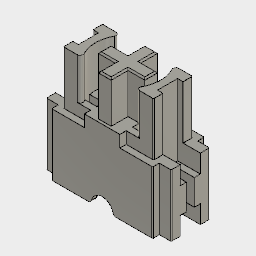
ALPS to MX stem (Autodesk Fusion 360 design; units mm, degrees)
Autodesk Fusion 360 part; units mm, degrees
sketch "Sketch1" plane through (0, 0, 0) normal (0, 0, 1) x (1, 0, 0)
  line L0 (0, 0) -> (10.7188, 0)
  line L1 (10.7188, 0) -> (10.7188, 4.445)
  line L2 (10.7188, 4.445) -> (0, 4.445)
  line L3 (0, 4.445) -> (0, 0)
  line L4 (0, 4.445) -> (1.016, 4.445)
  line L5 (1.016, 4.445) -> (1.016, 3.8735)
  line L6 (1.016, 3.8735) -> (0, 3.8735)
  line L7 (0, 3.8735) -> (0, 4.445)
  line L8 (0, 0) -> (1.016, 0)
  line L9 (1.016, 0) -> (1.016, 0.5715)
  line L10 (1.016, 0.5715) -> (0, 0.5715)
  line L11 (0, 0.5715) -> (0, 0)
  line L12 (10.7188, 4.445) -> (9.7028, 4.445)
  line L13 (9.7028, 4.445) -> (9.7028, 3.8735)
  line L14 (9.7028, 3.8735) -> (10.7188, 3.8735)
  line L15 (10.7188, 3.8735) -> (10.7188, 4.445)
  line L16 (10.7188, 0) -> (9.7028, 0)
  line L17 (9.7028, 0) -> (9.7028, 0.5715)
  line L18 (9.7028, 0.5715) -> (10.7188, 0.5715)
  line L19 (10.7188, 0.5715) -> (10.7188, 0)
  line L20 (5.3594, 4.445) -> (5.3594, 0) construction
  line L21 (0, 2.2225) -> (10.7188, 2.2225) construction
  line L22 (0, 3.0861) -> (1.9558, 3.0861)
  line L23 (1.9558, 3.0861) -> (1.9558, 1.3589)
  line L24 (1.9558, 1.3589) -> (0, 1.3589)
  line L25 (0, 1.3589) -> (0, 3.0861)
  line L26 (8.763, 3.0861) -> (10.7188, 3.0861)
  line L27 (10.7188, 3.0861) -> (10.7188, 1.3589)
  line L28 (10.7188, 1.3589) -> (8.763, 1.3589)
  line L29 (8.763, 1.3589) -> (8.763, 3.0861)
  circle A0 centre (5.3594, 2.2225) radius 1.0922
  circle A1 centre (5.3594, 2.2225) radius 1.905
  line L30 (1.9558, 3.0861) -> (2.5908, 3.0861)
  line L31 (2.5908, 3.0861) -> (2.5908, 1.3589)
  line L32 (2.5908, 1.3589) -> (1.9558, 1.3589)
  line L33 (1.9558, 1.3589) -> (1.9558, 3.0861)
  line L34 (8.763, 3.0861) -> (8.128, 3.0861)
  line L35 (8.128, 3.0861) -> (8.128, 1.3589)
  line L36 (8.128, 1.3589) -> (8.763, 1.3589)
  line L37 (8.763, 1.3589) -> (8.763, 3.0861)
  line L38 (2.5908, 3.3655) -> (3.8354, 3.3655)
  line L39 (3.8354, 3.3655) -> (3.8354, 1.0795)
  line L40 (3.8354, 1.0795) -> (2.5908, 1.0795)
  line L41 (2.5908, 1.0795) -> (2.5908, 3.3655)
  line L42 (8.128, 3.3655) -> (6.8834, 3.3655)
  line L43 (6.8834, 3.3655) -> (6.8834, 1.0795)
  line L44 (6.8834, 1.0795) -> (8.128, 1.0795)
  line L45 (8.128, 1.0795) -> (8.128, 3.3655)
  dimension "d1" = 4.445
  dimension "d2" = 10.7188
  dimension "d3" = 3.302
  dimension "d4" = 1.7272
  dimension "d5" = 8.6868
  dimension "d6" = 6.8072
  dimension "d7" = 2.1844
  dimension "d8" = 3.81
  dimension "d10" = 0.635
  dimension "d12" = 2.286
  measures "d1" distance of L0.start L2.end
  measures "d2" distance of L1.end L2.end
  measures "d3" distance of L6 L10
  measures "d4" distance of L22.end L23.end
  measures "d5" distance of L5 L13
  measures "d6" distance of L23 L29
  measures "d7" diameter of A0
  measures "d8" diameter of A1
  measures "d10" distance of L22.end L30.end
  measures "d12" distance of L38.start L40.end
extrude "Extrude1" add sketch "Sketch1" along normal blind 5.334 contours L0 L1 L3 L9 L10 L17 L18 L24 L28 A1 L32 L36 L40 L41 L44 L45 | L1 L2 L3 L5 L6 L13 L14 L22 L26 A1 L30 L34 L38 L41 L42 L45 | L23 L30 L31 L32 L33 L41 | L29 L34 L35 L36 L37 L45 | A0 makes body 1 at (6.4502, 2.1681, 3.556) makes body 2 at (3.9116, 4.445, 3.556)
sketch "Sketch2" plane through (0, 0, 0) normal (-1, 0, 0) x (0, -1, 0)
  line L0 (-1.3589, 0) -> (-0.5715, 0) construction
  line L1 (-0.5715, 0) -> (-0.5715, 5.334) construction
  line L2 (-0.5715, 5.334) -> (-1.3589, 5.334) construction
  line L3 (-1.3589, 5.334) -> (-1.3589, 0) construction
  line L4 (-1.3589, 5.334) -> (-0.5715, 5.334) construction
  line L5 (-3.8735, 5.334) -> (-3.0861, 5.334) construction
  line L6 (-3.8735, 5.334) -> (-3.0861, 5.334) construction
  line L7 (-3.0861, 5.334) -> (-3.0861, 0) construction
  line L8 (-3.0861, 0) -> (-3.8735, 0) construction
  line L9 (-3.8735, 0) -> (-3.8735, 5.334) construction
  line L10 (-1.3589, 5.334) -> (-0.5715, 5.334) construction
  line L11 (-0.5715, 5.334) -> (-0.5715, 0) construction
  line L12 (-0.5715, 0) -> (-1.3589, 0) construction
  line L13 (-1.3589, 0) -> (-1.3589, 5.334) construction
  line L14 (-3.8735, 2.667) -> (-0.5715, 2.667) construction
  line L15 (-3.0861, 3.7719) -> (-2.5654, 3.7719)
  line L16 (-2.5654, 3.7719) -> (-2.5654, 1.5621)
  line L17 (-2.5654, 1.5621) -> (-3.0861, 1.5621)
  line L18 (-3.0861, 1.5621) -> (-3.0861, 3.7719)
  line L19 (-1.3589, 3.7719) -> (-1.8796, 3.7719)
  line L20 (-1.8796, 3.7719) -> (-1.8796, 1.5621)
  line L21 (-1.8796, 1.5621) -> (-1.3589, 1.5621)
  line L22 (-1.3589, 1.5621) -> (-1.3589, 3.7719)
  point P0 (-3.0861, 0)
  dimension "d16" = 2.2098
  dimension "d17" = 0.6858
  dimension "d18" = 1.3081
  measures "d16" distance of L15 L17
  measures "d17" distance of L16 L20
  measures "d18" distance of L9 L16
extrude "Extrude2" add sketch "Sketch2" against normal up to surface (1.9558 mm away) bodies 2
sketch "Sketch3" plane through (10.7188, 0, 0) normal (1, 0, 0) x (0, 1, 0)
  line L0 (0.5715, 0) -> (1.3589, 0)
  line L1 (1.3589, 0) -> (1.3589, 5.334)
  line L2 (1.3589, 5.334) -> (0.5715, 5.334)
  line L3 (0.5715, 5.334) -> (0.5715, 0)
  line L4 (3.8735, 0) -> (3.0861, 0)
  line L5 (3.0861, 0) -> (3.0861, 1.5621)
  line L6 (3.0861, 1.5621) -> (2.5654, 1.5621)
  line L7 (2.5654, 1.5621) -> (2.5654, 3.7719)
  line L8 (2.5654, 3.7719) -> (3.0861, 3.7719)
  line L9 (3.0861, 3.7719) -> (3.0861, 5.334)
  line L10 (3.0861, 5.334) -> (3.8735, 5.334)
  line L11 (3.8735, 5.334) -> (3.8735, 0)
  line L12 (1.3589, 0) -> (0.5715, 0)
  line L13 (0.5715, 0) -> (0.5715, 5.334)
  line L14 (0.5715, 5.334) -> (1.3589, 5.334)
  line L15 (1.3589, 5.334) -> (1.3589, 3.7719)
  line L16 (1.3589, 3.7719) -> (1.8796, 3.7719)
  line L17 (1.8796, 3.7719) -> (1.8796, 1.5621)
  line L18 (1.8796, 1.5621) -> (1.3589, 1.5621)
  line L19 (1.3589, 1.5621) -> (1.3589, 0)
  line L20 (3.0861, 3.7719) -> (3.0861, 1.5621)
  line L21 (1.3589, 3.7719) -> (1.3589, 1.5621)
extrude "Extrude3" add sketch "Sketch3" against normal up to surface (1.9558 mm away) contours L1 L16 L17 L18 L21 | L6 L7 L8 L20 bodies 2
sketch "Sketch4" plane through (0, 0, 5.334) normal (0, 0, 1) x (-1, 0, 0)
  arc A0 (-3.8354, -1.0795) -> (-6.8834, -1.0795) centre (-5.3594, -2.2225) ccw
  line L0 (-3.8354, -1.0795) -> (-2.5908, -1.0795)
  line L1 (-2.5908, -1.0795) -> (-2.5908, -3.3655)
  line L2 (-2.5908, -3.3655) -> (-3.8354, -3.3655)
  arc A1 (-6.8834, -3.3655) -> (-3.8354, -3.3655) centre (-5.3594, -2.2225) ccw
  line L3 (-6.8834, -3.3655) -> (-8.128, -3.3655)
  line L4 (-8.128, -3.3655) -> (-8.128, -1.0795)
  line L5 (-8.128, -1.0795) -> (-6.8834, -1.0795)
  line L6 (-1.016, 0) -> (-9.7028, 0)
  line L7 (-9.7028, 0) -> (-9.7028, -0.5715)
  line L8 (-9.7028, -0.5715) -> (-10.7188, -0.5715)
  line L9 (-10.7188, -0.5715) -> (-10.7188, -1.3589)
  line L10 (-10.7188, -1.3589) -> (-8.763, -1.3589)
  line L11 (-8.763, -1.3589) -> (-8.763, -3.0861)
  line L12 (-8.763, -3.0861) -> (-10.7188, -3.0861)
  line L13 (-10.7188, -3.0861) -> (-10.7188, -3.8735)
  line L14 (-10.7188, -3.8735) -> (-9.7028, -3.8735)
  line L15 (-9.7028, -3.8735) -> (-9.7028, -4.445)
  line L16 (-9.7028, -4.445) -> (-1.016, -4.445)
  line L17 (-1.016, -4.445) -> (-1.016, -3.8735)
  line L18 (-1.016, -3.8735) -> (0, -3.8735)
  line L19 (0, -3.8735) -> (0, -3.0861)
  line L20 (0, -3.0861) -> (-1.9558, -3.0861)
  line L21 (-1.9558, -3.0861) -> (-1.9558, -1.3589)
  line L22 (-1.9558, -1.3589) -> (0, -1.3589)
  line L23 (0, -1.3589) -> (0, -0.5715)
  line L24 (0, -0.5715) -> (-1.016, -0.5715)
  line L25 (-1.016, -0.5715) -> (-1.016, 0)
  circle A2 centre (-5.3594, -2.2225) radius 1.0922
  line L26 (-5.9055, -4.2164) -> (-4.8133, -4.2164)
  line L27 (-4.8133, -4.2164) -> (-4.8133, -0.2286)
  line L28 (-4.8133, -0.2286) -> (-5.9055, -0.2286)
  line L29 (-5.9055, -0.2286) -> (-5.9055, -4.2164)
  line L30 (-5.9055, -4.2164) -> (-4.8133, -0.2286) construction
  line L31 (-4.8133, -4.2164) -> (-5.9055, -0.2286) construction
  line L32 (-7.3533, -2.7686) -> (-3.3655, -2.7686)
  line L33 (-3.3655, -2.7686) -> (-3.3655, -1.6764)
  line L34 (-3.3655, -1.6764) -> (-7.3533, -1.6764)
  line L35 (-7.3533, -1.6764) -> (-7.3533, -2.7686)
  line L36 (-7.3533, -2.7686) -> (-3.3655, -1.6764) construction
  line L37 (-3.3655, -2.7686) -> (-7.3533, -1.6764) construction
  line L38 (-6.8834, -4.445) -> (-3.8354, -4.445)
  line L39 (-3.8354, -4.445) -> (-3.8354, 0)
  line L40 (-3.8354, 0) -> (-6.8834, 0)
  line L41 (-6.8834, 0) -> (-6.8834, -4.445)
  line L42 (-6.8834, -4.445) -> (-3.8354, 0) construction
  line L43 (-3.8354, -4.445) -> (-6.8834, 0) construction
  line L44 (-3.3655, -2.7686) -> (-1.9558, -2.7686)
  line L45 (-1.9558, -2.7686) -> (-1.9558, -1.6764)
  line L46 (-1.9558, -1.6764) -> (-3.3655, -1.6764)
  line L47 (-3.3655, -1.6764) -> (-3.3655, -2.7686)
  line L48 (-7.3533, -2.7686) -> (-8.763, -2.7686)
  line L49 (-8.763, -2.7686) -> (-8.763, -1.6764)
  line L50 (-8.763, -1.6764) -> (-7.3533, -1.6764)
  line L51 (-7.3533, -1.6764) -> (-7.3533, -2.7686)
  point P0 (-5.3594, -2.2225)
  point P1 (-5.3594, -2.2225)
  point P2 (-5.3594, -2.2225)
  dimension "d23" = 1.0922
  dimension "d25" = 3.9878
  measures "d23" distance of L26.start L26.end
  measures "d25" distance of L26.start L28.end
extrude "Extrude4" add sketch "Sketch4" along normal blind 1.016 contours A0 A2 L27 L34 L39 | A0 L6 L27 L28 L29 L39 L40 L41 | A0 A2 L27 L29 | A0 L27 L28 L29 | A2 L32 L34 L39 | L32 L33 L34 L39 L47 | A0 A2 L29 L34 L41 | A2 L27 L29 L34 | A2 L27 L34 | L1 L21 L44 L45 L46 | L1 L33 L44 L46 L47 | A2 L27 L32 L34 | A1 A2 L27 L32 L39 | A2 L29 L34 | L27 L29 L32 L34 | A2 L27 L32 | A1 L16 L26 L27 L29 L38 L39 L41 | L32 L34 L35 L41 L51 | A2 L32 L34 L41 | A2 L29 L32 L34 | A2 L27 L29 L32 | A1 A2 L27 L29 | A1 L26 L27 L29 | L4 L35 L48 L50 L51 | L4 L11 L48 L49 L50 | A1 A2 L29 L32 L41 | A2 L29 L32 bodies 1 2
sketch "Sketch5" plane through (0, 0, 6.35) normal (0, 0, 1) x (-1, 0, 0)
  line L0 (-6.8834, 0) -> (-6.8834, -1.6764)
  line L1 (-6.8834, -4.445) -> (-3.8354, -4.445)
  line L2 (-3.8354, -4.445) -> (-3.8354, -2.7686)
  line L3 (-3.8354, 0) -> (-6.8834, 0)
  line L4 (-3.3655, -2.7686) -> (-3.3655, -1.6764)
  line L5 (-7.3533, -2.7686) -> (-3.3655, -2.7686)
  line L6 (-3.3655, -1.6764) -> (-7.3533, -1.6764)
  line L7 (-7.3533, -1.6764) -> (-7.3533, -2.7686)
  line L8 (-5.9055, -0.2286) -> (-5.9055, -4.2164)
  line L9 (-5.9055, -4.2164) -> (-4.8133, -4.2164)
  line L10 (-4.8133, -4.2164) -> (-4.8133, -0.2286)
  line L11 (-4.8133, -0.2286) -> (-5.9055, -0.2286)
  line L12 (-6.8834, -1.6764) -> (-8.763, -1.6764)
  line L13 (-8.763, -2.7686) -> (-6.8834, -2.7686)
  line L14 (-6.8834, -2.7686) -> (-6.8834, -4.445)
  line L15 (-3.8354, -2.7686) -> (-1.9558, -2.7686)
  line L16 (-1.9558, -1.6764) -> (-3.8354, -1.6764)
  line L17 (-3.8354, -1.6764) -> (-3.8354, 0)
  line L18 (-1.9558, -2.7686) -> (-1.9558, -1.6764)
  line L19 (-8.763, -1.6764) -> (-8.763, -2.7686)
extrude "Extrude5" add sketch "Sketch5" along normal blind 3.556 contours L5 L6 L7 L8 L12 L13 | L6 L8 L10 L11 | L5 L6 L8 L10 | L4 L5 L6 L10 L15 L16 | L5 L8 L9 L10 bodies 1
sketch "Sketch6" plane through (0, 0, 5.334) normal (0, 0, 1) x (-1, 0, 0)
  line L0 (-8.763, -1.6764) -> (-8.128, -1.6764)
  line L1 (-8.128, -1.6764) -> (-8.128, -1.0795)
  line L2 (-8.128, -1.0795) -> (-6.8834, -1.0795)
  line L3 (-6.8834, -1.0795) -> (-6.8834, 0)
  line L4 (-6.8834, 0) -> (-9.7028, 0)
  line L5 (-9.7028, 0) -> (-9.7028, -0.5715)
  line L6 (-9.7028, -0.5715) -> (-10.7188, -0.5715)
  line L7 (-10.7188, -0.5715) -> (-10.7188, -1.3589)
  line L8 (-10.7188, -1.3589) -> (-8.763, -1.3589)
  line L9 (-8.763, -1.3589) -> (-8.763, -1.6764)
  line L10 (-6.8834, -4.445) -> (-6.8834, -3.3655)
  line L11 (-6.8834, -3.3655) -> (-8.128, -3.3655)
  line L12 (-8.128, -3.3655) -> (-8.128, -2.7686)
  line L13 (-8.128, -2.7686) -> (-8.763, -2.7686)
  line L14 (-8.763, -2.7686) -> (-8.763, -3.0861)
  line L15 (-8.763, -3.0861) -> (-10.7188, -3.0861)
  line L16 (-10.7188, -3.0861) -> (-10.7188, -3.8735)
  line L17 (-10.7188, -3.8735) -> (-9.7028, -3.8735)
  line L18 (-9.7028, -3.8735) -> (-9.7028, -4.445)
  line L19 (-9.7028, -4.445) -> (-6.8834, -4.445)
  arc A0 (-3.8354, -1.0795) -> (-6.8834, -1.0795) centre (-5.3594, -2.2225) ccw
  line L20 (-6.8834, -1.0795) -> (-8.128, -1.0795)
  line L21 (-8.128, -1.0795) -> (-8.128, -3.3655)
  line L22 (-8.128, -3.3655) -> (-6.8834, -3.3655)
  arc A1 (-6.8834, -3.3655) -> (-3.8354, -3.3655) centre (-5.3594, -2.2225) ccw
  line L23 (-3.8354, -3.3655) -> (-2.5908, -3.3655)
  line L24 (-2.5908, -3.3655) -> (-2.5908, -1.0795)
  line L25 (-2.5908, -1.0795) -> (-3.8354, -1.0795)
  line L26 (-9.7028, 0) -> (-1.016, 0)
  line L27 (-1.016, 0) -> (-1.016, -0.5715)
  line L28 (-1.016, -0.5715) -> (0, -0.5715)
  line L29 (0, -0.5715) -> (0, -1.3589)
  line L30 (0, -1.3589) -> (-1.9558, -1.3589)
  line L31 (-1.9558, -1.3589) -> (-1.9558, -3.0861)
  line L32 (-1.9558, -3.0861) -> (0, -3.0861)
  line L33 (0, -3.0861) -> (0, -3.8735)
  line L34 (0, -3.8735) -> (-1.016, -3.8735)
  line L35 (-1.016, -3.8735) -> (-1.016, -4.445)
  line L36 (-1.016, -4.445) -> (-9.7028, -4.445)
  line L37 (-9.7028, -4.445) -> (-9.7028, -3.8735)
  line L38 (-9.7028, -3.8735) -> (-10.7188, -3.8735)
  line L39 (-10.7188, -3.8735) -> (-10.7188, -3.0861)
  line L40 (-10.7188, -3.0861) -> (-8.763, -3.0861)
  line L41 (-8.763, -3.0861) -> (-8.763, -1.3589)
  line L42 (-8.763, -1.3589) -> (-10.7188, -1.3589)
  line L43 (-10.7188, -1.3589) -> (-10.7188, -0.5715)
  line L44 (-10.7188, -0.5715) -> (-9.7028, -0.5715)
  line L45 (-9.7028, -0.5715) -> (-9.7028, 0)
  line L46 (-5.3594, -4.445) -> (-5.3594, 0) construction
  line L47 (-1.9558, -2.2225) -> (-8.763, -2.2225) construction
  line L48 (-9.2329, -3.8989) -> (-1.4859, -3.8989)
  line L49 (-1.4859, -3.8989) -> (-1.4859, -0.5461)
  line L50 (-1.4859, -0.5461) -> (-9.2329, -0.5461)
  line L51 (-9.2329, -0.5461) -> (-9.2329, -3.8989)
  line L52 (-9.2329, -3.8989) -> (-1.4859, -0.5461) construction
  line L53 (-1.4859, -3.8989) -> (-9.2329, -0.5461) construction
  line L54 (-1.4859, -3.0861) -> (-1.9558, -3.0861)
  line L55 (-1.9558, -3.0861) -> (-1.9558, -1.3589)
  line L56 (-1.9558, -1.3589) -> (-1.4859, -1.3589)
  line L57 (-1.4859, -1.3589) -> (-1.4859, -3.0861)
  circle A2 centre (-5.3594, -2.2225) radius 2.794
  point P0 (-5.3594, -2.2225)
  dimension "d30" = 7.747
  dimension "d31" = 3.3528
  dimension "d32" = 5.588
  measures "d30" distance of L48.start L48.end
  measures "d31" distance of L48.end L49.end
  measures "d32" diameter of A2
extrude "Extrude6" add sketch "Sketch6" along normal up to surface (4.572 mm away) contours L0 L1 L2 L8 L9 L20 L21 L41 L42 L50 L51 A2 | L0 L13 L21 L41 A2 | L1 L2 L20 L21 A2 | L11 L12 L13 L14 L15 L21 L22 L40 L41 L48 L51 A2 | L11 L12 L21 L22 A2 | L23 L24 L25 L30 L31 L32 L48 L49 L50 L54 L55 L56 A2 | L24 L25 A2 | L23 L24 A2 bodies 1
extrude "Extrude7" add sketch "Sketch6" along normal up to surface (1.016 mm away) contours L2 L3 L20 L50 A2 | L10 L11 L22 L48 A2 | A0 L25 L50 A2 | A1 L23 L48 A2 bodies 1
chamfer "Chamfer1" distance 0.127 angle 45 12 edges at (5.3594, 0.2286, 9.906) (3.3655, 2.2225, 9.906) (5.3594, 4.2164, 9.906) (7.3533, 2.2225, 9.906) (6.6294, 1.6764, 9.906) (5.9055, 0.9525, 9.906) (4.8133, 0.9525, 9.906) (4.0894, 1.6764, 9.906) (4.0894, 2.7686, 9.906) (4.8133, 3.4925, 9.906) (5.9055, 3.4925, 9.906) (6.6294, 2.7686, 9.906) on bodies 1
fillet "Fillet1" radius 0.254 4 edges at (3.1242, 0.5461, 8.128) (3.1242, 3.8989, 8.128) (7.5946, 0.5461, 8.128) (7.5946, 3.8989, 8.128) on bodies 1
fillet "Fillet2" radius 0.0762 16 edges at (1.4859, 3.0861, 7.62) (1.4859, 3.8989, 7.62) (1.4859, 1.3589, 7.62) (1.4859, 0.5461, 7.62) (9.2329, 0.5461, 7.62) (9.2329, 1.3589, 7.62) (9.2329, 3.0861, 7.62) (9.2329, 3.8989, 7.62) (1.016, 0, 2.667) (0, 0.5715, 2.667) (0, 3.8735, 2.667) (9.7028, 0, 2.667) (10.7188, 0.5715, 2.667) (10.7188, 3.8735, 2.667) (9.7028, 4.445, 2.667) (1.016, 4.445, 2.667) on bodies 1
fillet "Fillet3" radius 0.127 1 edges at (4.3411, 1.8275, 0) on bodies 1
sketch "Sketch7" plane through (0, 0, 0) normal (0, 0, -1) x (1, 0, 0)
  arc A0 (1.016, -4.3688) -> (1.0922, -4.445) centre (1.0922, -4.3688) ccw
  line L0 (1.0922, -4.445) -> (9.6266, -4.445)
  arc A1 (9.6266, -4.445) -> (9.7028, -4.3688) centre (9.6266, -4.3688) ccw
  line L1 (9.7028, -4.3688) -> (9.7028, -3.8735)
  line L2 (9.7028, -3.8735) -> (10.6426, -3.8735)
  arc A2 (10.6426, -3.8735) -> (10.7188, -3.7973) centre (10.6426, -3.7973) ccw
  line L3 (10.7188, -3.7973) -> (10.7188, -3.0861)
  line L4 (10.7188, -3.0861) -> (8.763, -3.0861)
  line L5 (8.763, -3.0861) -> (8.763, -1.3589)
  line L6 (8.763, -1.3589) -> (10.7188, -1.3589)
  line L7 (10.7188, -1.3589) -> (10.7188, -0.6477)
  arc A3 (10.7188, -0.6477) -> (10.6426, -0.5715) centre (10.6426, -0.6477) ccw
  line L8 (10.6426, -0.5715) -> (9.7028, -0.5715)
  line L9 (9.7028, -0.5715) -> (9.7028, -0.0762)
  arc A4 (9.7028, -0.0762) -> (9.6266, 0) centre (9.6266, -0.0762) ccw
  line L10 (9.6266, 0) -> (1.0922, 0)
  arc A5 (1.0922, 0) -> (1.016, -0.0762) centre (1.0922, -0.0762) ccw
  line L11 (1.016, -0.0762) -> (1.016, -0.5715)
  line L12 (1.016, -0.5715) -> (0.0762, -0.5715)
  arc A6 (0.0762, -0.5715) -> (0, -0.6477) centre (0.0762, -0.6477) ccw
  line L13 (0, -0.6477) -> (0, -1.3589)
  line L14 (0, -1.3589) -> (1.9558, -1.3589)
  line L15 (1.9558, -1.3589) -> (1.9558, -3.0861)
  line L16 (1.9558, -3.0861) -> (0, -3.0861)
  line L17 (0, -3.0861) -> (0, -3.7973)
  arc A7 (0, -3.7973) -> (0.0762, -3.8735) centre (0.0762, -3.7973) ccw
  line L18 (0.0762, -3.8735) -> (1.016, -3.8735)
  line L19 (1.016, -3.8735) -> (1.016, -4.3688)
  arc A8 (6.8834, -1.0795) -> (3.8354, -1.0795) centre (5.3594, -2.2225) ccw
  line L20 (6.8834, -1.0795) -> (8.128, -1.0795)
  line L21 (8.128, -1.0795) -> (8.128, -3.3655)
  line L22 (8.128, -3.3655) -> (6.8834, -3.3655)
  arc A9 (3.8354, -3.3655) -> (6.8834, -3.3655) centre (5.3594, -2.2225) ccw
  line L23 (3.8354, -3.3655) -> (2.5908, -3.3655)
  line L24 (2.5908, -3.3655) -> (2.5908, -1.0795)
  line L25 (2.5908, -1.0795) -> (3.8354, -1.0795)
  line L26 (6.3119, 0) -> (4.4069, 0)
  line L27 (4.4069, 0) -> (4.4069, -4.445)
  line L28 (4.4069, -4.445) -> (6.3119, -4.445)
  line L29 (6.3119, -4.445) -> (6.3119, 0)
  line L30 (6.3119, 0) -> (4.4069, -4.445) construction
  line L31 (4.4069, 0) -> (6.3119, -4.445) construction
  point P0 (5.3594, -2.2225)
  dimension "d42" = 1.905
  measures "d42" distance of L26.start L26.end
sketch "Sketch8" plane through (0, 4.445, 0) normal (0, 1, 0) x (-1, 0, 0)
  line L0 (-1.0922, 0) -> (-1.0922, 5.334)
  line L1 (-1.0922, 5.334) -> (-3.8354, 5.334)
  line L2 (-3.8354, 5.334) -> (-3.8354, 6.35)
  line L3 (-3.8354, 6.35) -> (-6.8834, 6.35)
  line L4 (-6.8834, 6.35) -> (-6.8834, 5.334)
  line L5 (-6.8834, 5.334) -> (-9.6266, 5.334)
  line L6 (-9.6266, 5.334) -> (-9.6266, 0)
  line L7 (-9.6266, 0) -> (-1.0922, 0)
  line L8 (-4.4069, 0) -> (-6.3119, 0)
  circle A0 centre (-5.3594, 0) radius 0.9525
  point P0 (-6.3119, 0)
extrude "Extrude8" cut sketch "Sketch8" against normal blind 0.762 contours L7 L8 A0 picked at (-5.1267, 0.216) bodies 1
sketch "Sketch9" plane through (0, 0, 0) normal (0, -1, 0) x (1, 0, 0)
  line L0 (9.6266, 0) -> (9.6266, 5.334)
  line L1 (9.6266, 5.334) -> (6.8834, 5.334)
  line L2 (6.8834, 5.334) -> (6.8834, 6.35)
  line L3 (6.8834, 6.35) -> (3.8354, 6.35)
  line L4 (3.8354, 6.35) -> (3.8354, 5.334)
  line L5 (3.8354, 5.334) -> (1.0922, 5.334)
  line L6 (1.0922, 5.334) -> (1.0922, 0)
  line L7 (1.0922, 0) -> (9.6266, 0)
  circle A0 centre (5.3594, 0) radius 0.9525
  point P0 (5.3594, 0)
  point P1 (6.3119, 0)
extrude "Extrude9" cut sketch "Sketch9" against normal blind 0.762 contours L7 A0 picked at (5.5921, 0.216) bodies 1
fillet "Fillet4" radius 0.254 4 edges at (6.3119, 0.2864, 0) (4.4069, 0.2864, 0) (4.4069, 4.1586, 0) (6.3119, 4.1586, 0) on bodies 1
fillet "Fillet5" radius 0.254 10 edges at (3.9962, 3.5532, 0) (4.3313, 3.8263, 0.0501) (5.3594, 4.1275, 0.9525) (6.3875, 3.8263, 0.0501) (6.7226, 3.5532, 0) (3.9962, 0.8918, 0) (4.3313, 0.6187, 0.0501) (5.3594, 0.3175, 0.9525) (6.3875, 0.6187, 0.0501) (6.7226, 0.8918, 0) on bodies 1
ref_plane "WorkPlane1" through (0.9779, 2.2225, 2.667) normal (0, -1, 0) x (0, 0, -1)
sketch "Sketch10" plane through (0.9779, 2.2225, 2.667) normal (0, -1, 0) x (1, 0, 0)
  line L0 (5.4737, 2.667) -> (3.2893, 2.667)
  line L1 (3.2893, -2.54) -> (5.4737, -2.54)
  line L2 (7.1501, -2.667) -> (7.1501, 2.667)
  line L3 (1.6129, -2.667) -> (1.6129, 2.667)
  line L4 (1.6129, 2.667) -> (1.6129, -2.667)
  line L5 (5.4737, 2.667) -> (7.1501, 2.2178)
  line L6 (3.2893, 2.667) -> (1.6129, 2.2178)
  line L7 (2.8575, 2.667) -> (1.6414, 2.667)
  line L8 (5.9055, 2.667) -> (7.1216, 2.667)
  line L9 (7.1501, 2.2178) -> (7.1501, 2.667)
  line L10 (5.4737, 2.667) -> (7.1501, 2.667)
  line L11 (3.2893, 2.667) -> (1.6129, 2.667)
  line L12 (1.6129, 2.667) -> (1.6129, 2.2178)
  dimension "d50" = 15
  dimension "d51" = 15
  measures "d50" angle of L6 L7
  measures "d51" angle of L5 L8
extrude "Extrude10" add sketch "Sketch10" against normal up to surface (0.5461 mm away) bodies 1
extrude "Extrude11" add sketch "Sketch10" along normal up to surface (0.5461 mm away) bodies 1
sketch "Sketch11" plane through (0.9779, 2.2225, 2.667) normal (0, -1, 0) x (1, 0, 0)
  line L0 (5.3467, -2.667) -> (3.4163, -2.667)
  line L1 (3.8354, 3.683) -> (4.9276, 3.683)
  line L2 (4.3815, -2.667) -> (4.3815, 3.683)
  line L3 (5.4737, 2.667) -> (3.2893, 2.667)
  line L4 (5.4737, 2.667) -> (4.3815, 2.667)
  line L5 (5.4737, 2.667) -> (7.1501, 2.2178)
  line L6 (7.1501, 2.2178) -> (7.1501, 2.667)
  line L7 (5.4737, 2.667) -> (7.1501, 2.667)
  point P0 (5.4737, 2.667)
  point P1 (7.1501, 2.2178)
  point P2 (7.1501, 2.667)
revolve "Revolve1" add sketch "Sketch11" angle 360 about axis through (5.3594, 2.2225, 0) along (0, 0, 1) bodies 1
sketch "Sketch12" plane through (0, 0, 6.35) normal (0, 0, 1) x (-1, 0, 0)
  line L0 (-3.8354, -3.3655) -> (-3.8354, -2.7686)
  line L1 (-3.8354, -2.7686) -> (-4.8133, -2.7686)
  line L2 (-4.8133, -2.7686) -> (-4.8133, -4.2164)
  line L3 (-4.8133, -4.2164) -> (-5.9055, -4.2164)
  line L4 (-5.9055, -4.2164) -> (-5.9055, -2.7686)
  line L5 (-5.9055, -2.7686) -> (-6.8834, -2.7686)
  line L6 (-6.8834, -2.7686) -> (-6.8834, -3.3655)
  line L7 (-6.8834, -3.3655) -> (-7.9089, -3.3655)
  arc A0 (-7.9089, -3.3655) -> (-7.8305, -3.5264) centre (-5.3594, -2.2225) ccw
  arc A1 (-8.0552, -3.8989) -> (-7.8305, -3.5264) centre (-8.0552, -3.6449) ccw
  line L8 (-8.0552, -3.8989) -> (-6.8834, -3.8989)
  line L9 (-6.8834, -3.8989) -> (-6.8834, -4.445)
  line L10 (-6.8834, -4.445) -> (-3.8354, -4.445)
  line L11 (-3.8354, -4.445) -> (-3.8354, -3.8989)
  line L12 (-3.8354, -3.8989) -> (-2.6636, -3.8989)
  arc A2 (-2.8883, -3.5264) -> (-2.6636, -3.8989) centre (-2.6636, -3.6449) ccw
  arc A3 (-2.8883, -3.5264) -> (-2.8099, -3.3655) centre (-5.3594, -2.2225) ccw
  line L13 (-2.8099, -3.3655) -> (-3.8354, -3.3655)
  line L14 (-7.0104, -4.445) -> (-3.7084, -4.445)
  line L15 (-3.7084, -4.445) -> (-4.4036, -5.6488)
  line L16 (-4.4036, -5.6488) -> (-6.7183, -5.144)
  line L17 (-6.7183, -5.144) -> (-7.0104, -4.445)
  line L18 (-7.0104, 0) -> (-3.7084, 0)
  line L19 (-3.7084, 0) -> (-4.461, 1.2734)
  line L20 (-4.461, 1.2734) -> (-6.7183, 1.0448)
  line L21 (-6.7183, 1.0448) -> (-7.0104, 0)
  line L22 (-6.8834, -1.0795) -> (-7.881, -1.0795)
  arc A4 (-7.881, -1.0795) -> (-8.0736, -1.6764) centre (-5.3594, -2.2225) ccw
  line L23 (-8.0736, -1.6764) -> (-6.8834, -1.6764)
  line L24 (-6.8834, -1.6764) -> (-6.8834, -1.0795)
  line L25 (-7.881, -3.3655) -> (-6.8834, -3.3655)
  line L26 (-6.8834, -3.3655) -> (-6.8834, -2.7686)
  line L27 (-6.8834, -2.7686) -> (-8.0736, -2.7686)
  arc A5 (-8.0736, -2.7686) -> (-7.881, -3.3655) centre (-5.3594, -2.2225) ccw
  line L28 (-2.6452, -2.7686) -> (-3.8354, -2.7686)
  line L29 (-3.8354, -2.7686) -> (-3.8354, -3.3655)
  line L30 (-3.8354, -3.3655) -> (-2.8378, -3.3655)
  arc A6 (-2.8378, -3.3655) -> (-2.6452, -2.7686) centre (-5.3594, -2.2225) ccw
  line L31 (-2.8378, -1.0795) -> (-3.8354, -1.0795)
  line L32 (-3.8354, -1.0795) -> (-3.8354, -1.6764)
  line L33 (-3.8354, -1.6764) -> (-2.6452, -1.6764)
  arc A7 (-2.6452, -1.6764) -> (-2.8378, -1.0795) centre (-5.3594, -2.2225) ccw
  point P0 (-7.0104, -4.445)
  point P1 (-3.7084, -4.445)
  point P2 (-7.0104, -4.445)
  point P3 (-7.0104, 0)
  point P4 (-3.7084, 0)
extrude "Extrude12" cut sketch "Sketch12" against normal blind 7.874 contours L0 L13 L28 L29 L30 A6 | L6 L7 L25 L26 L27 A5 | L10 L14 L15 L16 L17 | L18 L19 L20 L21 | L22 A4 L23 L24 | L31 L32 L33 A7 bodies 1
fillet "Fillet6" radius 0.254 4 edges at (8.021, 1.3726, 5.334) (8.021, 3.0724, 5.334) (2.6978, 3.0724, 5.334) (2.6978, 1.3726, 5.334) on bodies 1
equation "d51 = d50"
